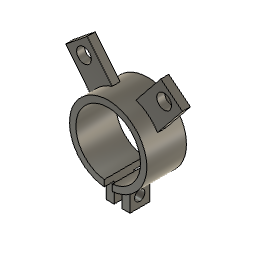
Steering bracket v2 (Autodesk Fusion 360 design; units mm, degrees)
Autodesk Fusion 360 part; units mm, degrees
sketch "Sketch2" plane through (0, 0, 0) normal (0, 1, 0) x (1, 0, 0)
  line L0 (0, -49.53) -> (-49.53, -49.53) construction
  line L1 (-49.53, -49.53) -> (-49.53, 0) construction
  line L2 (-49.53, 0) -> (0, 0) construction
  line L3 (0, 0) -> (0, -49.53) construction
  circle A0 centre (-24.765, -24.765) radius 24.765
  line L4 (0, -24.765) -> (-49.53, -24.765)
  line L5 (-24.765, -49.53) -> (-24.765, 0)
  circle A1 centre (-24.765, -24.765) radius 20.701
  line L6 (-27.305, -49.53) -> (-27.305, -0.1306) construction
  line L7 (-22.225, -49.3994) -> (-22.225, -0.1306) construction
  line L8 (-27.305, -0.1306) -> (-32.385, -0.1306)
  line L9 (-32.385, -0.1306) -> (-32.385, 12.5694)
  line L10 (-32.385, 12.5694) -> (-27.305, 12.5694)
  line L11 (-27.305, 12.5694) -> (-27.305, -0.1306)
  line L12 (-22.225, -0.1306) -> (-17.145, -0.1306)
  line L13 (-17.145, -0.1306) -> (-17.145, 12.5694)
  line L14 (-17.145, 12.5694) -> (-22.225, 12.5694)
  line L15 (-22.225, 12.5694) -> (-22.225, -0.1306)
  line L16 (-17.145, -0.1306) -> (-17.145, -1.2015)
  line L17 (-32.385, -0.1306) -> (-32.385, -1.2015)
  line L18 (0, -37.1475) -> (-49.53, -37.1475)
  line L19 (-46.2121, -37.1475) -> (-32.3872, -48.3278)
  line L20 (-32.3872, -48.3278) -> (-48.3591, -68.0777)
  line L21 (-48.3591, -68.0777) -> (-62.184, -56.8974)
  line L22 (-62.184, -56.8974) -> (-46.2121, -37.1475)
  line L23 (-39.2997, -42.7377) -> (-55.2716, -62.4876)
  line L24 (-1.1709, -68.0777) -> (12.654, -56.8974)
  line L25 (-17.1428, -48.3278) -> (-1.1709, -68.0777)
  line L26 (12.654, -56.8974) -> (-3.3179, -37.1475)
  line L27 (-3.3179, -37.1475) -> (-17.1428, -48.3278)
  line L28 (-27.305, -4.2204) -> (-27.305, -0.1306)
  line L29 (-22.225, -4.2204) -> (-22.225, -0.1306)
  line L30 (-57.3925, -50.9724) -> (-43.5675, -62.1528) construction
  circle A2 centre (-50.48, -56.5626) radius 4.7244
  circle A3 centre (0.95, -56.5626) radius 4.7244
  line L31 (34.0291, -75.6602) -> (-92.9709, -75.6602)
  line L32 (-92.9709, -75.6602) -> (-92.9709, -50.2602)
  line L33 (-92.9709, -50.2602) -> (34.0291, -50.2602)
  line L34 (34.0291, -50.2602) -> (34.0291, -75.6602)
  dimension "d68" = 49.53
  dimension "d69" = 49.53
  dimension "d70" = 49.53
  dimension "d71" = 41.402
  dimension "d72" = 5.08
  dimension "d73" = 5.08
  dimension "d74" = 12.7
  dimension "d75" = 5.08
  dimension "d76" = 5.08
  dimension "d77" = 12.7
  dimension "d82" = 12.3825
  dimension "d85" = 17.78
  dimension "d87" = 25.4
  dimension "d88" = 24.765
  dimension "d119" = 7.62
  dimension "d120" = 9.4488
  dimension "d124" = 25.4
  dimension "d125" = 127
  constraint horizontal L0
  constraint vertical L1
  constraint horizontal L2
  constraint vertical L3
  constraint coincident L2.end L3.start
  constraint midpoint L3 L4.start
  constraint midpoint L1 L4.end
  constraint midpoint L0 L5.start
  constraint midpoint L2 L5.end
  constraint midpoint A0.centre L5
  constraint concentric A0 A1
  constraint coincident L0 L6.start
  constraint coincident A0 L6.end
  constraint perpendicular L2 L6
  constraint coincident A0 L7.start
  constraint coincident A0 L7.end
  constraint perpendicular L2 L7
  constraint horizontal L8
  constraint vertical L9
  constraint horizontal L10
  constraint vertical L11
  constraint horizontal L12
  constraint vertical L13
  constraint horizontal L14
  constraint vertical L15
  constraint coincident A0 L16.end
  constraint perpendicular L12 L16
  constraint coincident A0 L17.end
  constraint perpendicular L8 L17
  constraint coincident L3 L18.start
  constraint coincident L1 L18.end
  constraint perpendicular L1 L18
  constraint perpendicular L19 L20
  constraint parallel L19 L21
  constraint parallel L20 L22
  constraint coincident L18 L19.start
  constraint coincident A0 L19.start
  constraint midpoint L19 L23.start
  constraint midpoint L21 L23.end
  constraint symmetric L5 L19.start L26.end
  constraint symmetric L5 L19.end L25.start
  constraint symmetric L5 L20.end L24.start
  constraint symmetric L5 L21.end L24.end
  constraint coincident A1 L28.start
  constraint coincident L6 L28.start
  constraint coincident L7 L29.start
  constraint coincident A1 L29.start
  constraint coincident L22 L30.start
  constraint coincident L20 L30.end
  constraint perpendicular L20 L30
  constraint midpoint L30 A2.centre
  constraint symmetric L5 A2 A3
  constraint horizontal L31
  constraint vertical L32
  constraint horizontal L33
  constraint vertical L34
  measures "d68" distance of L0.start L0.end
  measures "d69" distance of L0.start L2.end
  measures "d70" diameter of A0
  measures "d71" diameter of A1
  measures "d74" distance of L6.end L10.end
  measures "d75" distance of L9.end L10.end
  measures "d76" distance of L7.end L12.end
  measures "d77" distance of L7.end L14.end
  measures "d82" distance of A0.centre L18
  measures "d85" distance of L19.start L19.end
  measures "d87" distance of L19.start L21.end
  measures "d88" distance of A0.centre L19.end
  measures "d119" distance of L21 L30
  measures "d120" diameter of A2
  measures "d124" distance of L31.start L33.end
  measures "d125" distance of L31.start L31.end
extrude "Extrude13" add sketch "Sketch2" along normal blind 2.54 contours A0 L25 L26 L33 | L24 L25 L26 L33 | A0 L20 L23 L33 | L20 L21 L23 A2 L33 | A0 L22 L23 L33 | L21 L22 L23 A2 L33 | L23 A2 | L23 A2 | A3 makes body 1 at (1.2205, 0, 55.9339) makes body 2 at (-49.8087, 0, 56.6956)
extrude "Extrude14" add sketch "Sketch2" against normal blind 2.54 contours A0 L25 L26 L33 | L24 L25 L26 L33 | A0 L20 L23 L33 | L20 L21 L23 A2 L33 | A0 L22 L23 L33 | L21 L22 L23 A2 L33 | L23 A2 | L23 A2 | A3 bodies 1 2
extrude "Extrude20" add sketch "Sketch2" along normal blind 12.7 contours A0 L4 A1 L29 | A0 L4 A1 L18 | A0 L5 A1 L18 L27 | A0 L27 | A0 L5 A1 L18 L19 | A0 L4 A1 L18 | A0 L4 A1 L28 | A0 L19 L23 | A0 L19 L23 bodies 1 2
extrude "Extrude21" add sketch "Sketch2" against normal blind 12.7 separate body contours A0 L4 A1 L29 | A0 L4 A1 L18 | A0 L5 A1 L18 L27 | A0 L5 A1 L18 L19 | A0 L4 A1 L18 | A0 L4 A1 L28 | A0 L19 L23 | A0 L19 L23 makes body 3
extrude "Extrude22" cut sketch "Sketch2" against normal blind 12.7 contours A0 L27 | A0 L19 L23 | A0 L19 L23 bodies 3
extrude "Extrude23" add sketch "Sketch2" against normal blind 12.7 contours A0 L27 | A0 L19 L23 | A0 L19 L23 bodies 1 3
extrude "Extrude18" add sketch "Sketch2" along normal blind 6.35 contours A0 L12 L16 | L12 L13 L14 L15 | A0 L8 L17 | L8 L9 L10 L11 bodies 1
extrude "Extrude19" add sketch "Sketch2" against normal blind 6.35 contours A0 L12 L16 | L12 L13 L14 L15 | A0 L8 L17 | L8 L9 L10 L11 bodies 1
hole "Hole4" at (-32.385, -0.1159, -5.7836) direction (1, 0, 0) diameter 0.2794 depth 3.81 tip angle 180 bodies 1
thread "Thread3" "ANSI Unified Screw Threads 0.0138 35-282 UNM 2B" major diameter 0.3556 minor diameter 0.2769 pitch 0.0901 angle 60 resizes the face on face at (-31.115, -0.2293, -5.7021) on bodies 1
hole "Hole5" at (-32.385, -0.1159, -5.7836) direction (1, 0, 0) diameter 6.604 depth 17.78 tip angle 180 bodies 1
delete_face "DeleteFace2" 1 faces at (1.2205, -2.54, 55.9339) on bodies 1
delete_face "DeleteFace3" 1 faces at (-49.8087, -2.54, 56.6956) on bodies 1
extrude "Extrude24" add sketch "Sketch2" along normal blind 2.54 contours A0 L25 L26 L33 | L24 L25 L26 L33 | A0 L20 L23 L33 | L20 L21 L23 A2 L33 | A0 L22 L23 L33 | L21 L22 L23 A2 L33 bodies 1
move_face "OffsetFaces1" offset 2.54 2 faces at (-42.3233, 0, 58.3393) (-7.2067, 0, 58.3393) on bodies 1
equation "d82 = ( 1.95 / 4 ) * 1 in"
equation "d88 = ( 1.95 / 2 ) * 1 in"
